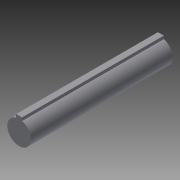
# Autodesk Inventor part: GearShaft
Saved by Autodesk Inventor 2015 SP1 (Build 190203100, 203)
## iProperties
Created: 2016-02-24
Part Number: GearShaft
Material: Generic
Document SubType Name: Modeling
Designer: jonesdm
Density: 1 g/cm^3
Appearance: Default
GearShaftL: 6.000 in
Author: jonesdm
Autodesk Inventor part; units mm, degrees
ref_plane "YZ Plane" through (0, 0, 0) normal (1, 0, 0) x (0, 1, 0)
ref_plane "XZ Plane" through (0, 0, 0) normal (0, 1, 0) x (-1, 0, 0)
ref_plane "XY Plane" through (0, 0, 0) normal (0, 0, 1) x (1, 0, 0)
sketch "Sketch1" plane through (0, 0, 0) normal (0, 0, 1) x (1, 0, 0)
  circle A0 centre (0, 0) radius 12.7
  line L0 (-3.175, 12.2967) -> (-3.175, 15.5987)
  line L1 (-3.175, 15.5987) -> (3.175, 15.5987)
  line L2 (3.175, 15.5987) -> (3.175, 12.2967)
  point P0 (0, 15.5987)
  dimension "d0" = 25.4
  dimension "d1" = 6.35
  dimension "d2" = 3.302
  constraints: 6 end point, 2 perpendicular, 2 point on circle, 1 centre point, 1 coincident, 1 midpoint, 1 vertical, 1 vertical alignment
  measures "d0" diameter of A0
  measures "d1" distance of L0.end L1.end
  measures "d2" distance of L1.end L2.end
extrude "Extrusion1" add sketch "Sketch1" along normal blind 152.4
equation "\"d3\" = GearShaftL"
equation "\"GearShaftL\" = 152.4"
body "Solid1"
